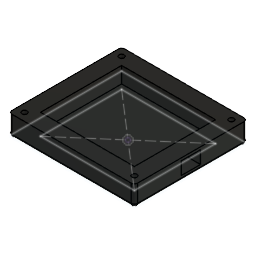
Macropad offical - Taksh Nahata (Autodesk Fusion 360 archive; units mm, degrees)
design "Bottom Case"
part number: 2026-05-30-17-30-41-830
Autodesk Fusion 360 part; units mm, degrees
sketch "Sketch1" plane through (0, 0, 0) normal (0, 0, 1) x (1, 0, 0)
  line L0 (29.4, 25.4) -> (-29.4, 25.4)
  line L1 (-29.4, 25.4) -> (-29.4, -25.4)
  line L2 (-29.4, -25.4) -> (29.4, -25.4)
  line L3 (29.4, -25.4) -> (29.4, 25.4)
  line L4 (29.4, 25.4) -> (-29.4, -25.4) construction
  line L5 (-29.4, 25.4) -> (29.4, -25.4) construction
  line L6 (-39.4, 35.4) -> (-39.4, -35.4)
  line L7 (-39.4, -35.4) -> (39.4, -35.4)
  line L8 (39.4, -35.4) -> (39.4, 35.4)
  line L9 (39.4, 35.4) -> (-39.4, 35.4)
  dimension "d1" = 58.8
  dimension "d2" = 50.8
  dimension "d3" = 10
  constraint horizontal L0
  constraint perpendicular L0 L1
  constraint parallel L0 L2
  constraint parallel L1 L3
  constraint coincident L4 origin
  constraint coincident L5 origin
  measures "d1" distance of L1.end L2.end
  measures "d2" distance of L0.end L1.end
extrude "Extrude6" add sketch "Sketch1" along normal blind 3 contours L0 L1 L2 L3
extrude "Extrude7" add sketch "Sketch1" along normal blind 13
sketch "Sketch2" plane through (39.4, 0, 0) normal (1, 0, 0) x (0, 1, 0)
  line L0 (-35.4, 0) -> (35.4, 0)
  line L1 (35.4, 0) -> (35.4, 13)
  line L2 (35.4, 13) -> (-35.4, 13)
  line L3 (-35.4, 13) -> (-35.4, 0)
  line L4 (6, 11.3977) -> (-6, 11.3977)
  line L5 (-6, 11.3977) -> (-6, 3.3977)
  line L6 (-6, 3.3977) -> (6, 3.3977)
  line L7 (6, 3.3977) -> (6, 11.3977)
  line L8 (6, 11.3977) -> (-6, 3.3977) construction
  line L9 (-6, 11.3977) -> (6, 3.3977) construction
  point P0 (0, 7.3977)
  dimension "d18" = 12
  dimension "d19" = 8
  constraint horizontal L4
  constraint perpendicular L4 L5
  constraint parallel L4 L6
  constraint parallel L5 L7
  constraint coincident L8 P0
  constraint coincident L9 P0
  measures "d18" distance of L5.end L6.end
  measures "d19" distance of L4.end L5.end
extrude "Extrude8" cut sketch "Sketch2" against normal blind 10 contours L4 L5 L6 L7
sketch "Sketch3" plane through (0, 0, 13) normal (0, 0, 1) x (1, 0, 0)
  line L0 (29.4, 25.4) -> (29.4, -25.4)
  line L1 (29.4, -25.4) -> (-29.4, -25.4)
  line L2 (-29.4, -25.4) -> (-29.4, 25.4)
  line L3 (-29.4, 25.4) -> (29.4, 25.4)
  line L4 (39.4, 35.4) -> (-39.4, 35.4)
  line L5 (-39.4, 35.4) -> (-39.4, -35.4)
  line L6 (-39.4, -35.4) -> (39.4, -35.4)
  line L7 (39.4, -35.4) -> (39.4, 35.4)
  circle A0 centre (-34.4, 30.4) radius 1.6
  circle A1 centre (34.4, 30.4) radius 1.6
  circle A2 centre (-34.4, -30.4) radius 1.6
  circle A3 centre (34.4, -30.4) radius 1.6
extrude "Extrude9" cut sketch "Sketch3" against normal blind 13 contours A0 | A1 | A2 | A3
fillet "Fillet1" radius 2 8 edges at (39.4, 0, 0) (39.4, 35.4, 6.5) (39.4, -35.4, 6.5) (0, -35.4, 0) (-39.4, -35.4, 6.5) (-39.4, 0, 0) (-39.4, 35.4, 6.5) (0, 35.4, 0)

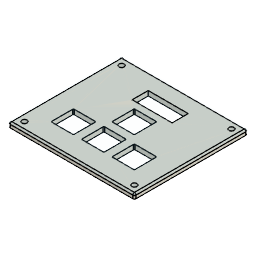
design "Top Plate"
part number: 2026-05-30-17-52-45-732
Autodesk Fusion 360 part; units mm, degrees
derive "DerivedContext1"
sketch "plate-2026-05-31T00_50_45.594Z" plane through (0, 0, 13) normal (0, 0, 1) x (1, 0, 0)
  line L0 (-6.425, 10.875) -> (6.575, 10.875)
  line L1 (-6.425, -3.125) -> (6.575, -3.125)
  line L2 (-6.925, 10.375) -> (-6.925, -2.625)
  line L3 (7.075, 10.375) -> (7.075, -2.625)
  arc A0 (-6.425, 10.875) -> (-6.925, 10.375) centre (-6.425, 10.375) ccw
  arc A1 (7.075, 10.375) -> (6.575, 10.875) centre (6.575, 10.375) ccw
  arc A2 (-6.925, -2.625) -> (-6.425, -3.125) centre (-6.425, -2.625) ccw
  arc A3 (6.575, -3.125) -> (7.075, -2.625) centre (6.575, -2.625) ccw
  line L4 (-25.475, -8.175) -> (-12.475, -8.175)
  line L5 (-25.475, -22.175) -> (-12.475, -22.175)
  line L6 (-25.975, -8.675) -> (-25.975, -21.675)
  line L7 (-11.975, -8.675) -> (-11.975, -21.675)
  arc A4 (-25.475, -8.175) -> (-25.975, -8.675) centre (-25.475, -8.675) ccw
  arc A5 (-11.975, -8.675) -> (-12.475, -8.175) centre (-12.475, -8.675) ccw
  arc A6 (-25.975, -21.675) -> (-25.475, -22.175) centre (-25.475, -21.675) ccw
  arc A7 (-12.475, -22.175) -> (-11.975, -21.675) centre (-12.475, -21.675) ccw
  line L8 (-6.425, -8.175) -> (6.575, -8.175)
  line L9 (-6.425, -22.175) -> (6.575, -22.175)
  line L10 (-6.925, -8.675) -> (-6.925, -21.675)
  line L11 (7.075, -8.675) -> (7.075, -21.675)
  arc A8 (-6.425, -8.175) -> (-6.925, -8.675) centre (-6.425, -8.675) ccw
  arc A9 (7.075, -8.675) -> (6.575, -8.175) centre (6.575, -8.675) ccw
  arc A10 (-6.925, -21.675) -> (-6.425, -22.175) centre (-6.425, -21.675) ccw
  arc A11 (6.575, -22.175) -> (7.075, -21.675) centre (6.575, -21.675) ccw
  line L12 (12.625, -8.175) -> (25.625, -8.175)
  line L13 (12.625, -22.175) -> (25.625, -22.175)
  line L14 (12.125, -8.675) -> (12.125, -21.675)
  line L15 (26.125, -8.675) -> (26.125, -21.675)
  arc A12 (12.625, -8.175) -> (12.125, -8.675) centre (12.625, -8.675) ccw
  arc A13 (26.125, -8.675) -> (25.625, -8.175) centre (25.625, -8.675) ccw
  arc A14 (12.125, -21.675) -> (12.625, -22.175) centre (12.625, -21.675) ccw
  arc A15 (25.625, -22.175) -> (26.125, -21.675) centre (25.625, -21.675) ccw
  line L16 (-28.5, -24.7) -> (28.65, -24.7)
  line L17 (-28.5, 13.4) -> (28.65, 13.4)
  line L18 (-28.5, -24.7) -> (-28.5, 13.4)
  line L19 (28.65, -24.7) -> (28.65, 13.4)
  line L20 (39.4, -35.4) -> (39.4, 35.4)
  line L21 (-39.4, -35.4) -> (39.4, -35.4)
  line L22 (39.4, 35.4) -> (-39.4, 35.4)
  line L23 (-39.4, 35.4) -> (-39.4, -35.4)
extrude "Extrude1" add sketch "plate-2026-05-31T00_50_45.594Z" along normal blind 3 contours L16 L17 L18 L19 | L20 L21 L22 L23
sketch "Sketch2" plane through (0, 0, 16) normal (0, 0, 1) x (-1, 0, 0)
  arc A0 (25.475, 8.175) -> (25.975, 8.675) centre (25.475, 8.675) ccw
  line L0 (25.475, 8.175) -> (12.475, 8.175)
  arc A1 (11.975, 8.675) -> (12.475, 8.175) centre (12.475, 8.675) ccw
  line L1 (11.975, 8.675) -> (11.975, 21.675)
  arc A2 (12.475, 22.175) -> (11.975, 21.675) centre (12.475, 21.675) ccw
  line L2 (12.475, 22.175) -> (25.475, 22.175)
  arc A3 (25.975, 21.675) -> (25.475, 22.175) centre (25.475, 21.675) ccw
  line L3 (25.975, 21.675) -> (25.975, 8.675)
  arc A4 (6.425, 8.175) -> (6.925, 8.675) centre (6.425, 8.675) ccw
  line L4 (6.425, 8.175) -> (-6.575, 8.175)
  arc A5 (-7.075, 8.675) -> (-6.575, 8.175) centre (-6.575, 8.675) ccw
  line L5 (-7.075, 8.675) -> (-7.075, 21.675)
  arc A6 (-6.575, 22.175) -> (-7.075, 21.675) centre (-6.575, 21.675) ccw
  line L6 (-6.575, 22.175) -> (6.425, 22.175)
  arc A7 (6.925, 21.675) -> (6.425, 22.175) centre (6.425, 21.675) ccw
  line L7 (6.925, 21.675) -> (6.925, 8.675)
  arc A8 (6.425, -10.875) -> (6.925, -10.375) centre (6.425, -10.375) ccw
  line L8 (6.425, -10.875) -> (-6.575, -10.875)
  arc A9 (-7.075, -10.375) -> (-6.575, -10.875) centre (-6.575, -10.375) ccw
  line L9 (-7.075, -10.375) -> (-7.075, 2.625)
  arc A10 (-6.575, 3.125) -> (-7.075, 2.625) centre (-6.575, 2.625) ccw
  line L10 (-6.575, 3.125) -> (6.425, 3.125)
  arc A11 (6.925, 2.625) -> (6.425, 3.125) centre (6.425, 2.625) ccw
  line L11 (6.925, 2.625) -> (6.925, -10.375)
  arc A12 (-12.625, 8.175) -> (-12.125, 8.675) centre (-12.625, 8.675) ccw
  line L12 (-12.625, 8.175) -> (-25.625, 8.175)
  arc A13 (-26.125, 8.675) -> (-25.625, 8.175) centre (-25.625, 8.675) ccw
  line L13 (-26.125, 8.675) -> (-26.125, 21.675)
  arc A14 (-25.625, 22.175) -> (-26.125, 21.675) centre (-25.625, 21.675) ccw
  line L14 (-25.625, 22.175) -> (-12.625, 22.175)
  arc A15 (-12.125, 21.675) -> (-12.625, 22.175) centre (-12.625, 21.675) ccw
  line L15 (-12.125, 21.675) -> (-12.125, 8.675)
  line L16 (39.4, -35.4) -> (39.4, 35.4)
  line L17 (39.4, 35.4) -> (-39.4, 35.4)
  line L18 (-39.4, 35.4) -> (-39.4, -35.4)
  line L19 (-39.4, -35.4) -> (39.4, -35.4)
sketch "Sketch7" plane through (0, 0, 16) normal (0, 0, 1) x (1, 0, 0)
  arc A0 (-25.475, -8.175) -> (-25.975, -8.675) centre (-25.475, -8.675) ccw
  line L0 (-25.475, -8.175) -> (-12.475, -8.175)
  arc A1 (-11.975, -8.675) -> (-12.475, -8.175) centre (-12.475, -8.675) ccw
  line L1 (-11.975, -8.675) -> (-11.975, -21.675)
  arc A2 (-12.475, -22.175) -> (-11.975, -21.675) centre (-12.475, -21.675) ccw
  line L2 (-12.475, -22.175) -> (-25.475, -22.175)
  arc A3 (-25.975, -21.675) -> (-25.475, -22.175) centre (-25.475, -21.675) ccw
  line L3 (-25.975, -21.675) -> (-25.975, -8.675)
  arc A4 (-6.425, -8.175) -> (-6.925, -8.675) centre (-6.425, -8.675) ccw
  line L4 (-6.425, -8.175) -> (6.575, -8.175)
  arc A5 (7.075, -8.675) -> (6.575, -8.175) centre (6.575, -8.675) ccw
  line L5 (7.075, -8.675) -> (7.075, -21.675)
  arc A6 (6.575, -22.175) -> (7.075, -21.675) centre (6.575, -21.675) ccw
  line L6 (6.575, -22.175) -> (-6.425, -22.175)
  arc A7 (-6.925, -21.675) -> (-6.425, -22.175) centre (-6.425, -21.675) ccw
  line L7 (-6.925, -21.675) -> (-6.925, -8.675)
  arc A8 (-6.425, 10.875) -> (-6.925, 10.375) centre (-6.425, 10.375) ccw
  line L8 (-6.425, 10.875) -> (6.575, 10.875)
  arc A9 (7.075, 10.375) -> (6.575, 10.875) centre (6.575, 10.375) ccw
  line L9 (7.075, 10.375) -> (7.075, -2.625)
  arc A10 (6.575, -3.125) -> (7.075, -2.625) centre (6.575, -2.625) ccw
  line L10 (6.575, -3.125) -> (-6.425, -3.125)
  arc A11 (-6.925, -2.625) -> (-6.425, -3.125) centre (-6.425, -2.625) ccw
  line L11 (-6.925, -2.625) -> (-6.925, 10.375)
  arc A12 (12.625, -8.175) -> (12.125, -8.675) centre (12.625, -8.675) ccw
  line L12 (12.625, -8.175) -> (25.625, -8.175)
  arc A13 (26.125, -8.675) -> (25.625, -8.175) centre (25.625, -8.675) ccw
  line L13 (26.125, -8.675) -> (26.125, -21.675)
  arc A14 (25.625, -22.175) -> (26.125, -21.675) centre (25.625, -21.675) ccw
  line L14 (25.625, -22.175) -> (12.625, -22.175)
  arc A15 (12.125, -21.675) -> (12.625, -22.175) centre (12.625, -21.675) ccw
  line L15 (12.125, -21.675) -> (12.125, -8.675)
  line L16 (-39.4, 35.4) -> (-39.4, -35.4)
  line L17 (-39.4, -35.4) -> (39.4, -35.4)
  line L18 (39.4, -35.4) -> (39.4, 35.4)
  line L19 (39.4, 35.4) -> (-39.4, 35.4)
  line L20 (-12.5, 15.14) -> (12.5, 15.14)
  line L21 (12.5, 15.14) -> (12.5, 25.14)
  line L22 (12.5, 25.14) -> (-12.5, 25.14)
  line L23 (-12.5, 25.14) -> (-12.5, 15.14)
extrude "Extrude3" cut sketch "Sketch7" against normal blind 3 contours L20 L21 L22 L23
sketch "Sketch8" plane through (0, 0, 16) normal (0, 0, 1) x (1, 0, 0)
  line L0 (12.5, 15.14) -> (-12.5, 15.14)
  line L1 (-12.5, 15.14) -> (-12.5, 25.14)
  line L2 (-12.5, 25.14) -> (12.5, 25.14)
  line L3 (12.5, 25.14) -> (12.5, 15.14)
  arc A0 (-6.425, 10.875) -> (-6.925, 10.375) centre (-6.425, 10.375) ccw
  line L4 (-6.425, 10.875) -> (6.575, 10.875)
  arc A1 (7.075, 10.375) -> (6.575, 10.875) centre (6.575, 10.375) ccw
  line L5 (7.075, 10.375) -> (7.075, -2.625)
  arc A2 (6.575, -3.125) -> (7.075, -2.625) centre (6.575, -2.625) ccw
  line L6 (6.575, -3.125) -> (-6.425, -3.125)
  arc A3 (-6.925, -2.625) -> (-6.425, -3.125) centre (-6.425, -2.625) ccw
  line L7 (-6.925, -2.625) -> (-6.925, 10.375)
  arc A4 (12.625, -8.175) -> (12.125, -8.675) centre (12.625, -8.675) ccw
  line L8 (12.625, -8.175) -> (25.625, -8.175)
  arc A5 (26.125, -8.675) -> (25.625, -8.175) centre (25.625, -8.675) ccw
  line L9 (26.125, -8.675) -> (26.125, -21.675)
  arc A6 (25.625, -22.175) -> (26.125, -21.675) centre (25.625, -21.675) ccw
  line L10 (25.625, -22.175) -> (12.625, -22.175)
  arc A7 (12.125, -21.675) -> (12.625, -22.175) centre (12.625, -21.675) ccw
  line L11 (12.125, -21.675) -> (12.125, -8.675)
  arc A8 (-6.425, -8.175) -> (-6.925, -8.675) centre (-6.425, -8.675) ccw
  line L12 (-6.425, -8.175) -> (6.575, -8.175)
  arc A9 (7.075, -8.675) -> (6.575, -8.175) centre (6.575, -8.675) ccw
  line L13 (7.075, -8.675) -> (7.075, -21.675)
  arc A10 (6.575, -22.175) -> (7.075, -21.675) centre (6.575, -21.675) ccw
  line L14 (6.575, -22.175) -> (-6.425, -22.175)
  arc A11 (-6.925, -21.675) -> (-6.425, -22.175) centre (-6.425, -21.675) ccw
  line L15 (-6.925, -21.675) -> (-6.925, -8.675)
  arc A12 (-25.475, -8.175) -> (-25.975, -8.675) centre (-25.475, -8.675) ccw
  line L16 (-25.475, -8.175) -> (-12.475, -8.175)
  arc A13 (-11.975, -8.675) -> (-12.475, -8.175) centre (-12.475, -8.675) ccw
  line L17 (-11.975, -8.675) -> (-11.975, -21.675)
  arc A14 (-12.475, -22.175) -> (-11.975, -21.675) centre (-12.475, -21.675) ccw
  line L18 (-12.475, -22.175) -> (-25.475, -22.175)
  arc A15 (-25.975, -21.675) -> (-25.475, -22.175) centre (-25.475, -21.675) ccw
  line L19 (-25.975, -21.675) -> (-25.975, -8.675)
  line L20 (-39.4, 35.4) -> (-39.4, -35.4)
  line L21 (-39.4, -35.4) -> (39.4, -35.4)
  line L22 (39.4, -35.4) -> (39.4, 35.4)
  line L23 (39.4, 35.4) -> (-39.4, 35.4)
  circle A16 centre (-34.4, 30.4) radius 1.6
  circle A17 centre (34.4, 30.4) radius 1.6
  circle A18 centre (-34.4, -30.4) radius 1.6
  circle A19 centre (34.4, -30.4) radius 1.6
extrude "Extrude4" cut sketch "Sketch8" against normal blind 16 contours A16 | A17 | A18 | A19
fillet "Fillet1" radius 1 8 edges at (-39.4, 35.4, 14.5) (0, 35.4, 16) (39.4, 35.4, 14.5) (39.4, 0, 16) (39.4, -35.4, 14.5) (0, -35.4, 16) (-39.4, -35.4, 14.5) (-39.4, 0, 16)
